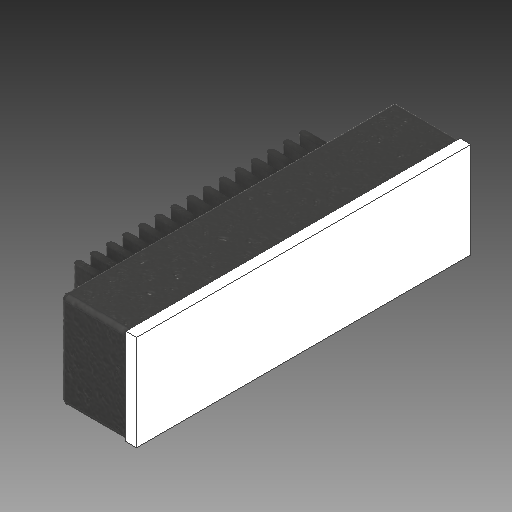
# Autodesk Inventor part: Bar Light Shruti
Saved by Autodesk Inventor 2019 (Build 230136000, 136)
## iProperties
Created: 2018-06-06
Part Number: Bar Light Shruti
Material: Generic
Document SubType Name: Modeling
Designer: Karthic
Density: 1 g/cm^3
Appearance: Default
Mass: 266.826 g
Surface Area: 539.686 cm^2
Volume: 266.826 cm^3
Author: Karthic
Autodesk Inventor part; units mm, degrees
ref_plane "YZ Plane" through (0, 0, 0) normal (1, 0, 0) x (0, 1, 0)
ref_plane "XZ Plane" through (0, 0, 0) normal (0, 1, 0) x (-1, 0, 0)
ref_plane "XY Plane" through (0, 0, 0) normal (0, 0, 1) x (1, 0, 0)
sketch "Sketch1" plane through (0, 0, 0) normal (0, 1, 0) x (-1, 0, 0)
  line L0 (15, 77) -> (-15, 77)
  line L1 (-15, 77) -> (-15, -77)
  line L2 (-15, -77) -> (15, -77)
  line L3 (15, -77) -> (15, 77)
  line L4 (15, 77) -> (-15, -77) construction
  line L5 (-15, 77) -> (15, -77) construction
  point P0 (0, 0)
  dimension "d0" = 154
  dimension "d1" = 30
  constraints: 12 end point, 2 midpoint, 2 parallel, 1 horizontal, 1 perpendicular
  measures "d0" distance of L2.end L0.start
  measures "d1" distance of L1.end L2.end
extrude "Extrusion1" add sketch "Sketch1" along normal blind 44
sketch "Sketch2" plane through (15, 0, 77) normal (1, 0, 0) x (0, 0, -1)
  line L0 (0, 44) -> (154, 44)
  line L1 (154, 44) -> (154, 0)
  line L2 (154, 0) -> (0, 0)
  line L3 (0, 0) -> (0, 44)
  line L4 (0, 0) -> (154, 0) projected
  line L5 (154, 0) -> (154, 44) projected
  line L6 (0, 44) -> (154, 44) projected
  line L7 (0, 0) -> (0, 44) projected
  point P0 (77, 0)
  constraints: 8 end point, 2 parallel, 1 horizontal, 1 perpendicular
sketch "Sketch3" plane through (-15, 0, -77) normal (0, 0, -1) x (-1, 0, 0)
  line L0 (-3.75, 25.567) -> (-1.0538, 19.1029)
  line L1 (-1.0538, 19.1029) -> (-5.3038, 13.5359)
  line L2 (-5.3038, 13.5359) -> (-12.25, 14.433)
  line L3 (-12.25, 14.433) -> (-14.9462, 20.8971)
  line L4 (-14.9462, 20.8971) -> (-10.6962, 26.4641)
  line L5 (-10.6962, 26.4641) -> (-3.75, 25.567)
  line L6 (0, 0) -> (0, 44) projected
  point P0 (-15, 0)
  point P1 (-8, 20)
  dimension "d66" = 8
  constraints: 12 end point, 13 other
  measures "d66" distance from line of L6 point (-8, 20)
extrude "Extrusion3" add sketch "Sketch3" along normal blind 2
sketch "Sketch4" plane through (-15, 0, -79) normal (0, 0, -1) x (-1, 0, 0)
  line L0 (-7, 27) -> (-1.1878, 23.067)
  line L1 (-1.1878, 23.067) -> (-1.6878, 16.067)
  line L2 (-1.6878, 16.067) -> (-8, 13)
  line L3 (-8, 13) -> (-13.8122, 16.933)
  line L4 (-13.8122, 16.933) -> (-13.3122, 23.933)
  line L5 (-13.3122, 23.933) -> (-7, 27)
  point P0 (-15, 0)
  point P1 (-7.5, 20)
  constraints: 12 end point, 13 other
extrude "Extrusion4" add sketch "Sketch4" along normal blind 2
sketch "Sketch5" plane through (-15, 0, -81) normal (0, 0, -1) x (-1, 0, 0)
  circle A0 centre (-7.5, 20) radius 6.0776
  point P0 (-15, 0)
  constraints: 1 centre point
extrude "Extrusion5" add sketch "Sketch5" along normal blind 1
sketch "Sketch6" plane through (-7.5, 20, -82) normal (0, 0, -1) x (-1, 0, 0)
  circle A0 centre (0, 0) radius 6.0776 projected
  circle A1 centre (0, 0) radius 5
  point P0 (-7.5, -20)
  constraints: 1 centre point, 1 coincident
extrude "Extrusion6" add sketch "Sketch6" along normal blind 5 contours A1
thread "Thread1" size "M10x1.5" class "6g" standard "ANSI Metric M Profile" full length
sketch "Sketch7" plane through (-7.5, 20, -87) normal (0, 0, -1) x (-1, 0, 0)
  circle A0 centre (0, 0) radius 5 projected
  circle A1 centre (0, 0) radius 4.5
  point P0 (-7.5, -20)
  dimension "d18" = 9
  constraints: 1 centre point, 1 coincident
  measures "d18" diameter of A1
extrude "Extrusion7" cut sketch "Sketch7" against normal up to surface (5 mm away) contours A1
sketch "Sketch8" plane through (-7.5, 20, -82) normal (0, 0, -1) x (-1, 0, 0)
  arc A0 (4.3875, -1) -> (4.3875, 1) centre (0, 0) ccw
  circle A1 centre (0, -2) radius 0.5
  circle A2 centre (0, 2) radius 0.5
  circle A3 centre (0, 0) radius 4.5 projected
  arc A4 (4.3875, 1) -> (4.3875, -1) centre (4.5, 0) ccw
  point P0 (-7.5, -20)
  dimension "d21" = 1
  dimension "d22" = 1
  dimension "d23" = 2
  dimension "d24" = 2
  constraints: 7 point on circle, 4 centre point
  measures "d21" diameter of A1
  measures "d22" diameter of A2
  measures "d23" distance of A0.centre A2.centre
  measures "d24" distance of A0.centre A1.centre
extrude "Extrusion8" add sketch "Sketch8" along normal up to surface (5 mm away) contours A4 A0 | A1 | A2
sketch "Sketch9" plane through (-15, 0, -77) normal (-1, 0, 0) x (0, 0, 1)
  line L0 (0, 0) -> (154, 0) projected
  line L1 (154, 0) -> (154, 44) projected
  line L2 (0, 44) -> (154, 44) projected
  line L3 (0, 0) -> (0, 44) projected
  circle A0 centre (11, 8.5) radius 2.8
  circle A1 centre (11, 8.5) radius 1.19
  circle A2 centre (11, 34.5) radius 2.8
  circle A3 centre (11, 34.5) radius 1.19
  circle A4 centre (143, 8.5) radius 2.8
  circle A5 centre (143, 8.5) radius 1.19
  circle A6 centre (143, 34.5) radius 2.8
  circle A7 centre (143, 34.5) radius 1.19
  point P0 (77, 0)
  dimension "d27" = 5.6
  dimension "d29" = 11
  dimension "d30" = 8.5
  dimension "d33" = 26
  dimension "d38" = 9.5
  dimension "d39" = 8.5
  dimension "d40" = 11
  dimension "d41" = 9.5
  dimension "d42" = 11
  dimension "d85" = 2.38
  dimension "d86" = 2.38
  dimension "d111" = 5.6
  dimension "d112" = 132
  dimension "d113" = 132
  dimension "d114" = 26
  dimension "d115" = 11
  dimension "d116" = 5.6
  dimension "d117" = 2.38
  dimension "d118" = 5.6
  dimension "d119" = 2.38
  constraints: 8 centre point, 1 horizontal alignment, 1 vertical, 3 other
  measures "d27" diameter of A0
  measures "d29" distance from line of L3 A0.centre
  measures "d30" distance from line of L0 A0.centre
  measures "d33" distance of A0.centre A2.centre
  measures "d38" distance from line of A2.centre L2
  measures "d39" distance from line of L0 A4.centre
  measures "d40" distance from line of L1 A4.centre
  measures "d41" distance from line of L2 A6.centre
  measures "d42" distance from line of L1 A6.centre
  measures "d85" diameter of A3
  measures "d86" diameter of A1
  measures "d111" diameter of A2
  measures "d112" distance of A4.centre A0.centre
  measures "d113" distance of A6.centre A2.centre
  measures "d114" distance of A6.centre A4.centre
  measures "d115" distance from line of L3 A2.centre
  measures "d116" diameter of A4
  measures "d117" diameter of A5
  measures "d118" diameter of A6
  measures "d119" diameter of A7
extrude "Extrusion9" add sketch "Sketch9" along normal blind 2.5 contours A0 | A2 | A4 | A6
thread "Thread2" size "M4x0.7" class "6H" standard "ANSI Metric M Profile" full length
thread "Thread3" size "M4x0.7" class "6H" standard "ANSI Metric M Profile" full length
thread "Thread4" size "M4x0.7" class "6H" standard "ANSI Metric M Profile" full length
thread "Thread5" size "M4x0.7" class "6H" standard "ANSI Metric M Profile" full length
sketch "Sketch10" plane through (-15, 0, -77) normal (-1, 0, 0) x (0, 0, 1)
  line L0 (0, 0) -> (0, 44) projected
  line L1 (21.5, 9.5) -> (131.5, 9.5)
  line L2 (131.5, 9.5) -> (131.5, 34.5)
  line L3 (131.5, 34.5) -> (21.5, 34.5)
  line L4 (21.5, 34.5) -> (21.5, 9.5)
  line L5 (21.5, 9.5) -> (131.5, 34.5) construction
  line L6 (131.5, 9.5) -> (21.5, 34.5) construction
  point P0 (77, 0)
  point P1 (76.5, 22)
  point P2 (0, 22)
  point P3 (76.5, 22)
  dimension "d53" = 110
  dimension "d54" = 25
  constraints: 12 end point, 4 midpoint, 2 parallel, 1 horizontal, 1 horizontal alignment, 1 perpendicular
  measures "d53" distance of L3.end L2.end
  measures "d54" distance of L3.end L1.start
extrude "Extrusion10" add sketch "Sketch10" along normal blind 5
sketch "Sketch11" plane through (-20, 0, -77) normal (-1, 0, 0) x (0, 0, 1)
  line L0 (131.5, 34.5) -> (21.5, 34.5) projected
  line L1 (21.5, 34.5) -> (21.5, 9.5) projected
  line L2 (131.5, 9.5) -> (21.5, 9.5) projected
  line L3 (23, 34.5) -> (26, 34.5)
  line L4 (26, 34.5) -> (26, 9.5)
  line L5 (26, 9.5) -> (23, 9.5)
  line L6 (23, 9.5) -> (23, 34.5)
  point P0 (77, 0)
  dimension "d57" = 1.5
  constraints: 8 end point, 2 parallel, 2 point on line, 1 horizontal, 1 perpendicular
  measures "d57" distance between parallel lines of L1 L6
extrude "Extrusion11" add sketch "Sketch11" along normal blind 14 contours L4 L2 L6 L0
pattern_linear "Rectangular Pattern1" count 15 spacing 7.4 along (0, 0, 1) of "Extrusion11"
fillet "Fillet2" radius 0.5 4 edges at (-17.5, 34.5, -68.8) (-17.5, 8.5, -68.8) (-17.5, 34.5, 63.2) (-17.5, 8.5, 63.2)
fillet "Fillet3" radius 1.5 30 edges at (-34, 22, -54) (-34, 22, -51) (-34, 22, -46.6) (-34, 22, -43.6) (-34, 22, -39.2) (-34, 22, -36.2) (-34, 22, -31.8) (-34, 22, -28.8) (-34, 22, -24.4) (-34, 22, -21.4) (-34, 22, -17) (-34, 22, -14) (-34, 22, -9.6) (-34, 22, -6.6) (-34, 22, -2.2) (-34, 22, 0.8) (-34, 22, 5.2) (-34, 22, 8.2) (-34, 22, 12.6) (-34, 22, 15.6) (-34, 22, 20) (-34, 22, 23) (-34, 22, 27.4) (-34, 22, 30.4) (-34, 22, 34.8) (-34, 22, 37.8) (-34, 22, 42.2) (-34, 22, 45.2) (-34, 22, 49.6) (-34, 22, 52.6)
sketch "Sketch12" plane through (15, 0, 77) normal (1, 0, 0) x (0, 0, -1)
  line L0 (154, 0) -> (154, 44) projected
  line L1 (0, 44) -> (154, 44)
  line L2 (154, 44) -> (154, 0)
  line L3 (154, 0) -> (0, 0)
  line L4 (0, 0) -> (0, 44)
  point P0 (77, 0)
  constraints: 8 end point, 2 parallel, 1 horizontal, 1 perpendicular
extrude "Extrusion12" add sketch "Sketch12" along normal blind 5 separate body
fillet "Fillet4" radius 2 7 edges at (0, 0, -77) (0, 44, -77) (0, 0, 77) (0, 44, 77) (-15, 44, 0) (-15, 22, 77) (-15, 0, 0)
sketch "Sketch14" plane through (-20, 0, -77) normal (-1, 0, 0) x (0, 0, 1)
  circle A0 centre (28.2, 21.5) radius 1.5 projected
  circle A1 centre (28.2, 21.5) radius 1.75
  point P0 (77, 0)
  dimension "d75" = 3.5
  constraints: 1 centre point, 1 coincident
  measures "d75" diameter of A1
extrude "Extrusion14" add sketch "Sketch14" along normal blind 1 contours A0 | A1 bodies 1
sketch "Sketch15" plane through (-21, 21.5, -48.8) normal (-1, 0, 0) x (0, 0, 1)
  line L0 (0, 1.3365) -> (0, -1) construction
  line L1 (-1.088, 0) -> (1, 0) construction
  line L2 (1.6771, 0.5) -> (0.5, 0.5)
  line L3 (-0.5, 0.5) -> (-1.6771, 0.5)
  line L4 (1.6771, -0.5) -> (0.5, -0.5)
  line L5 (-0.5, -0.5) -> (-1.6771, -0.5)
  line L6 (-0.5, -1.6771) -> (-0.5, -0.5)
  line L7 (-0.5, 0.5) -> (-0.5, 1.6771)
  line L8 (0.5, -1.6771) -> (0.5, -0.5)
  line L9 (0.5, 0.5) -> (0.5, 1.6771)
  circle A0 centre (0, 0) radius 1.75
  point P0 (48.8, -21.5)
  constraints: 20 end point, 4 symmetric about line, 2 horizontal, 2 vertical, 2 other
extrude "Extrusion15" cut sketch "Sketch15" against normal blind 0.5 contours A0 L4 L8 L6 L5 L3 L7 L9 L2 bodies 1
pattern_linear "Rectangular Pattern2" count 2 spacing 96 along (0, 0, 1) of "Extrusion15", "Extrusion14" bodies 1
fillet "Fillet5" radius 0.25 4 edges at (-15, 8.5, -68.8) (-15, 34.5, -68.8) (-15, 34.5, 63.2) (-15, 8.5, 63.2)
ref_plane "Work Plane1" through (0, 22, 0) normal (0, -1, 0) x (1, 0, 0)
body "Solid1"
body "Solid2"
